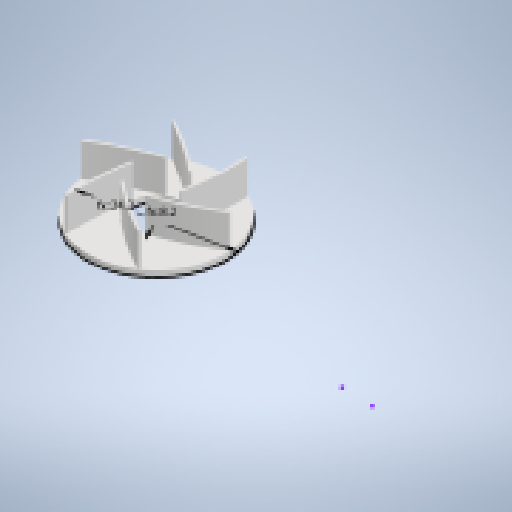
# Autodesk Inventor part: Propeller
Saved by Autodesk Inventor 2023.1 (Build 271208000, 208)
## iProperties
Created: 2024-02-14
Part Number: Propeller
Material: Generic
Document SubType Name: Modeling
Designer: USER
Density: 1 g/cm^3
Appearance: Default
Author: USER
Autodesk Inventor part; units mm, degrees
ref_plane "YZ Plane" through (0, 0, 0) normal (1, 0, 0) x (0, 1, 0)
ref_plane "XZ Plane" through (0, 0, 0) normal (0, 1, 0) x (-1, 0, 0)
ref_plane "XY Plane" through (0, 0, 0) normal (0, 0, 1) x (1, 0, 0)
sketch "Sketch1" plane through (0, 0, 0) normal (0, 1, 0) x (-1, 0, 0)
  circle A0 centre (0, 0) radius 12.1
  circle A1 centre (0, 0) radius 4.1
  arc A2 (4.1, 0) -> (4.8843, 10.8913) centre (-47.1092, 9.1614) ccw
  arc A3 (4.4623, -0.1893) -> (5.3321, 10.7237) centre (-41.6643, 8.9784) ccw
  line L0 (4.8843, 10.8913) -> (5.3321, 10.7237)
  line L1 (4.1, 0) -> (4.4623, -0.1893)
  dimension "d1" = 8.2
  dimension "d0" = 24.2
  constraints: 5 point on circle, 4 end point, 3 centre point, 2 coincident, 3 other
  measures "d0" diameter of A0
extrude "Extrusion1" add sketch "Sketch1" along normal blind 2
extrude "Extrusion2" add sketch "Sketch1" along normal blind 6.7625 contours A2 L0 A3 L1
pattern_circular "Circular Pattern1" count 6 over 360 about axis through (0, 0, 0) along (0, 1, 0) of "Extrusion2"
equation "\"d1\" = PropHoleDiameter"
equation "\"d0\" = PropDiameter"
equation "\"PropDiameter\" = 24.2"
equation "\"PropHoleDiameter\" = 8.2"
body "Solid1"
